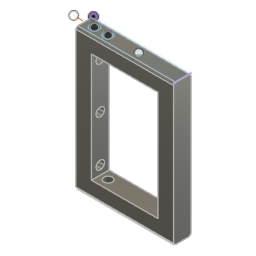
rear_chassis_brace (Autodesk Fusion 360 design; units mm, degrees)
Autodesk Fusion 360 part; units mm, degrees
sketch "Esquisse1" plane through (0, 0, 0) normal (0, 0, 1) x (1, 0, 0)
  line L0 (50, 0) -> (0, 0)
  line L1 (0, 0) -> (0, 72)
  line L2 (0, 72) -> (50, 72)
  line L3 (50, 72) -> (50, 0)
  line L4 (42, 64) -> (8, 64)
  line L5 (8, 64) -> (8, 8)
  line L6 (8, 8) -> (42, 8)
  line L7 (42, 8) -> (42, 64)
  dimension "d3" = 72
  dimension "d4" = 50
  dimension "d26" = 8
  dimension "d27" = 8
  dimension "d28" = 8
  dimension "d29" = 8
  constraint coincident L0.end L1.start
  constraint horizontal L0
  constraint perpendicular L0 L1
  constraint perpendicular L1 L2
  constraint perpendicular L0 L3
  constraint horizontal L4
  constraint vertical L5
  constraint horizontal L6
  constraint vertical L7
  measures "d3" distance of L0.end L1.end
  measures "d4" distance of L0.start L0.end
  measures "d26" distance of L0 L6
  measures "d27" distance of L1 L5
  measures "d28" distance of L3 L7
  measures "d29" distance of L2 L4
extrude "Extrusion1" add sketch "Esquisse1" along normal blind 9
sketch "Esquisse2" plane through (0, 0, 0) normal (0, -1, 0) x (1, 0, 0)
  line L0 (0, 0) -> (50, 0)
  line L1 (50, 9) -> (0, 9)
  line L2 (0, 9) -> (0, 0)
  line L3 (-5.7525, 4.5) -> (21.5406, 4.5) construction
  circle A0 centre (5, 4.5) radius 2.175
  circle A1 centre (12, 4.5) radius 2.175
  line L4 (50, 0) -> (50, 9)
  dimension "d7" = 4.35
  dimension "d8" = 7
  dimension "d9" = 4.5
  dimension "d10" = 5
  constraint coincident L3 A0.centre
  constraint coincident L3 A1.centre
  constraint equal A0 A1
  measures "d7" diameter of A0
  measures "d8" distance of A0.centre A1.centre
  measures "d9" vertical distance of L0.start L3.start
  measures "d10" distance of L2 A0.centre
extrude "Extrusion2" cut sketch "Esquisse2" against normal blind 8 contours A0 | A1
sketch "Esquisse3" plane through (0, 72, 0) normal (0, 1, 0) x (-1, 0, 0)
  line L0 (-50, 0) -> (0, 0)
  line L1 (0, 0) -> (0, 9)
  line L2 (0, 9) -> (-50, 9)
  line L3 (5.6122, 4.5) -> (-27.7174, 4.5) construction
  circle A0 centre (-12, 4.5) radius 2.175
  circle A1 centre (-5, 4.5) radius 2.175
  line L4 (-50, 9) -> (-50, 0)
  dimension "d13" = 4.5
  dimension "d14" = 7
  dimension "d15" = 5
  dimension "d16" = 4.35
  constraint coincident L3 A0.centre
  constraint coincident L3 A1.centre
  constraint equal A0 A1
  measures "d13" distance of L0.end L3
  measures "d14" distance of A0.centre A1.centre
  measures "d15" distance of L1 A1.centre
  measures "d16" diameter of A0
extrude "Extrusion3" cut sketch "Esquisse3" against normal blind 8 contours A0 | A1
sketch "Esquisse4" plane through (0, 0, 0) normal (-1, 0, 0) x (0, 0, 1)
  line L0 (0, 72) -> (0, 0)
  line L1 (0, 0) -> (9, 0)
  line L2 (9, 0) -> (9, 72)
  line L3 (9, 72) -> (0, 72)
  line L4 (4.5, 76) -> (4.5, -2) construction
  circle A0 centre (4.5, 12.5) radius 2.175
  circle A1 centre (4.5, 59.5) radius 2.175
  circle A2 centre (4.5, 36) radius 2.175
  dimension "d19" = 4.35
  dimension "d20" = 12.5
  dimension "d21" = 12.5
  dimension "d22" = 23.5
  dimension "d25" = 4.5
  constraint perpendicular L1 L4
  constraint coincident L4 A0.centre
  constraint coincident L4 A1.centre
  constraint equal A0 A1
  constraint coincident L4 A2.centre
  constraint equal A0 A2
  measures "d19" diameter of A0
  measures "d20" distance of L1 A0.centre
  measures "d21" distance of L3 A1.centre
  measures "d22" distance of A0.centre A2.centre
  measures "d25" distance of L0.end L4
extrude "Extrusion4" cut sketch "Esquisse4" against normal blind 8 contours A0 | A1 | A2
chamfer "Chanfrein1" distance 1 angle 45 4 edges at (25, 0, 9) (25, 72, 9) (25, 72, 0) (25, 0, 0)
equation "d21 = d20"
equation "d22 = ( 47 / 2 ) * 1 mm"
equation "d27 = d26"
equation "d28 = d26"
equation "d29 = d26"
